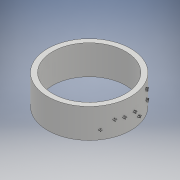
# Autodesk Inventor part: velky-vuz
Saved by Autodesk Inventor 2018 (Build 220112000, 112)
## iProperties
Created: 2019-09-09
Part Number: velky-vuz
Material: Generic
Document SubType Name: Modeling
Designer: dsikar
Density: 1 g/cm^3
Appearance: Default
Author: dsikar
Autodesk Inventor part; units mm, degrees
ref_plane "XZ Plane" through (0, 0, 0) normal (0, 1, 0) x (-1, 0, 0)
ref_plane "XY Plane" through (0, 0, 0) normal (0, 0, 1) x (1, 0, 0)
sketch "Sketch1" plane through (0, 0, 0) normal (0, 1, 0) x (-1, 0, 0)
  line L0 (8.7, 0) -> (9.9, 0)
  line L1 (9.9, 0) -> (9.9, 7)
  line L2 (9.9, 7) -> (8.7, 7)
  line L3 (8.7, 7) -> (8.7, 0)
  line L4 (0, -1.4) -> (0, 8.4) projected
  point P0 (0, 0)
  dimension "d0" = 1.2
  dimension "d1" = 7
  dimension "d2" = 8.7
  constraints: 8 end point, 2 parallel, 1 horizontal, 1 perpendicular
  measures "d0" distance of L2.end L1.end
  measures "d1" distance of L1.end L0.end
  measures "d2" distance from line of L3 point (0, 0)
revolve "Revolution1" add sketch "Sketch1" angle 360 about axis through (0, 0, -10) along (0, 0, 1)
ref_plane "Work Plane1" through (15, 0, 0) normal (1, 0, 0) x (0, 1, 0)
sketch "Sketch2" plane through (15, 0, 0) normal (1, 0, 0) x (0, 1, 0)
  line L0 (-6.8018, 10.1756) -> (6.3794, 10.1756) construction
  line L1 (6.3794, 10.1756) -> (6.3794, -3.0056) construction
  line L2 (6.3794, -3.0056) -> (-6.8018, -3.0056) construction
  line L3 (-6.8018, -3.0056) -> (-6.8018, 10.1756) construction
  line L4 (-5.9444, 2.3561) -> (-5.8589, 2.3561)
  line L5 (-5.8589, 1.9313) -> (-5.9444, 1.9313)
  line L6 (-5.6398, 2.2119) -> (-5.6398, 2.129)
  line L7 (-6.1956, 2.129) -> (-6.1956, 2.2119)
  line L8 (-3.4429, 4.0019) -> (-3.3959, 4.0019)
  line L9 (-3.3959, 3.4529) -> (-3.4429, 3.4529)
  line L10 (-3.0817, 3.7671) -> (-3.0817, 3.7274)
  line L11 (-3.721, 3.7274) -> (-3.721, 3.7671)
  line L12 (-1.532, 3.8011) -> (-1.483, 3.8011)
  line L13 (-1.483, 3.1927) -> (-1.532, 3.1927)
  line L14 (-1.1572, 3.556) -> (-1.1572, 3.51)
  line L15 (-1.829, 3.51) -> (-1.829, 3.556)
  line L16 (1.1865, 3.533) -> (1.1865, 3.4969)
  line L17 (0.5052, 3.4969) -> (0.5052, 3.533)
  line L18 (0.8159, 3.8011) -> (0.8688, 3.8011)
  line L19 (0.8688, 3.2117) -> (0.8159, 3.2117)
  line L20 (2.0208, 2.0898) -> (2.0975, 2.0898)
  line L21 (2.0975, 1.5943) -> (2.0208, 1.5943)
  line L22 (2.4219, 1.9313) -> (2.4219, 1.8421)
  line L23 (1.6905, 1.8421) -> (1.6905, 1.9313)
  line L24 (5.5222, 5.5708) -> (5.5222, 5.5026)
  line L25 (4.7754, 5.5026) -> (4.7754, 5.5708)
  line L26 (5.0253, 5.8028) -> (5.0939, 5.8028)
  line L27 (5.0939, 5.0977) -> (5.0253, 5.0977)
  line L28 (5.3072, 3.4529) -> (5.3766, 3.4529)
  line L29 (5.3766, 2.6743) -> (5.3072, 2.6743)
  line L30 (5.0253, 3.1061) -> (5.0253, 3.1927)
  line L31 (5.0253, 5.0977) -> (5.0253, 5.3948)
  line L32 (5.0253, 5.6103) -> (5.0253, 5.8028)
  line L33 (5.0939, 5.8028) -> (5.0939, 5.6303)
  line L34 (5.0939, 5.3748) -> (5.0939, 5.0977)
  arc A0 (4.9661, 5.5026) -> (5.0253, 5.3948) centre (5.0939, 5.5026) ccw
  arc A1 (5.0939, 5.3748) -> (5.2216, 5.5026) centre (5.0939, 5.5026) ccw
  line L35 (5.5222, 5.5026) -> (5.2216, 5.5026)
  line L36 (4.9661, 5.5026) -> (4.7754, 5.5026)
  line L37 (4.7754, 5.5708) -> (4.9859, 5.5708)
  line L38 (5.2018, 5.5708) -> (5.5222, 5.5708)
  arc A2 (5.2018, 5.5708) -> (5.0939, 5.6303) centre (5.0939, 5.5026) ccw
  arc A3 (5.0253, 5.6103) -> (4.9859, 5.5708) centre (5.0939, 5.5026) ccw
  line L39 (5.0253, 3.1927) -> (5.2596, 3.1927)
  line L40 (5.4936, 3.1927) -> (5.7458, 3.1927)
  line L41 (5.7458, 3.1061) -> (5.5222, 3.1061)
  line L42 (5.231, 3.1061) -> (5.0253, 3.1061)
  arc A4 (5.3072, 3.2341) -> (5.2596, 3.1927) centre (5.3766, 3.1061) ccw
  arc A5 (5.231, 3.1061) -> (5.3072, 2.9781) centre (5.3766, 3.1061) ccw
  line L43 (5.3072, 2.6743) -> (5.3072, 2.9781)
  line L44 (5.3072, 3.2341) -> (5.3072, 3.4529)
  line L45 (5.3766, 3.4529) -> (5.3766, 3.2517)
  line L46 (5.3766, 2.9605) -> (5.3766, 2.6743)
  arc A6 (5.3766, 2.9605) -> (5.5222, 3.1061) centre (5.3766, 3.1061) ccw
  arc A7 (5.4936, 3.1927) -> (5.3766, 3.2517) centre (5.3766, 3.1061) ccw
  line L47 (1.6905, 1.9313) -> (1.9625, 1.9313)
  line L48 (2.1667, 1.9313) -> (2.4219, 1.9313)
  line L49 (2.4219, 1.8421) -> (2.1823, 1.8421)
  line L50 (1.9469, 1.8421) -> (1.6905, 1.8421)
  arc A8 (2.0208, 1.9796) -> (1.9625, 1.9313) centre (2.0646, 1.8675) ccw
  arc A9 (1.9469, 1.8421) -> (2.0208, 1.7553) centre (2.0646, 1.8675) ccw
  line L51 (2.0208, 1.5943) -> (2.0208, 1.7553)
  line L52 (2.0208, 1.9796) -> (2.0208, 2.0898)
  line L53 (2.0975, 2.0898) -> (2.0975, 1.9833)
  line L54 (2.0975, 1.7516) -> (2.0975, 1.5943)
  arc A10 (2.0975, 1.7516) -> (2.1823, 1.8421) centre (2.0646, 1.8675) ccw
  arc A11 (2.1667, 1.9313) -> (2.0975, 1.9833) centre (2.0646, 1.8675) ccw
  line L55 (0.5052, 3.533) -> (0.6841, 3.533)
  line L56 (0.9948, 3.533) -> (1.1865, 3.533)
  line L57 (1.1865, 3.4969) -> (0.9959, 3.4969)
  line L58 (0.683, 3.4969) -> (0.5052, 3.4969)
  arc A12 (0.8159, 3.6652) -> (0.6841, 3.533) centre (0.8394, 3.51) ccw
  arc A13 (0.683, 3.4969) -> (0.8159, 3.3548) centre (0.8394, 3.51) ccw
  line L59 (0.8159, 3.2117) -> (0.8159, 3.3548)
  line L60 (0.8159, 3.6652) -> (0.8159, 3.8011)
  line L61 (0.8688, 3.8011) -> (0.8688, 3.6642)
  line L62 (0.8688, 3.3558) -> (0.8688, 3.2117)
  arc A14 (0.8688, 3.3558) -> (0.9959, 3.4969) centre (0.8394, 3.51) ccw
  arc A15 (0.9948, 3.533) -> (0.8688, 3.6642) centre (0.8394, 3.51) ccw
  line L63 (-1.1572, 3.51) -> (-1.3685, 3.51)
  line L64 (-1.6378, 3.51) -> (-1.829, 3.51)
  line L65 (-1.829, 3.556) -> (-1.6297, 3.556)
  line L66 (-1.3767, 3.556) -> (-1.1572, 3.556)
  arc A16 (-1.532, 3.6415) -> (-1.6297, 3.556) centre (-1.5032, 3.51) ccw
  arc A17 (-1.6378, 3.51) -> (-1.532, 3.3785) centre (-1.5032, 3.51) ccw
  line L67 (-1.532, 3.1927) -> (-1.532, 3.3785)
  line L68 (-1.532, 3.6415) -> (-1.532, 3.8011)
  line L69 (-1.483, 3.8011) -> (-1.483, 3.6431)
  line L70 (-1.483, 3.3769) -> (-1.483, 3.1927)
  arc A18 (-1.483, 3.3769) -> (-1.3685, 3.51) centre (-1.5032, 3.51) ccw
  arc A19 (-1.3767, 3.556) -> (-1.483, 3.6431) centre (-1.5032, 3.51) ccw
  line L71 (-3.3959, 4.0019) -> (-3.3959, 3.8762)
  line L72 (-3.4429, 3.8746) -> (-3.4429, 4.0019)
  line L73 (-3.721, 3.7671) -> (-3.5507, 3.7671)
  line L74 (-3.5531, 3.7274) -> (-3.721, 3.7274)
  line L75 (-3.4429, 3.4529) -> (-3.4429, 3.6031)
  line L76 (-3.3959, 3.6016) -> (-3.3959, 3.4529)
  line L77 (-3.0817, 3.7274) -> (-3.2768, 3.7274)
  line L78 (-3.2793, 3.7671) -> (-3.0817, 3.7671)
  arc A20 (-3.4429, 3.8746) -> (-3.5507, 3.7671) centre (-3.415, 3.7389) ccw
  arc A21 (-3.5531, 3.7274) -> (-3.4429, 3.6031) centre (-3.415, 3.7389) ccw
  arc A22 (-3.3959, 3.6016) -> (-3.2768, 3.7274) centre (-3.415, 3.7389) ccw
  arc A23 (-3.2793, 3.7671) -> (-3.3959, 3.8762) centre (-3.415, 3.7389) ccw
  line L79 (-5.6398, 2.129) -> (-5.7835, 2.129)
  line L80 (-6.0279, 2.129) -> (-6.1956, 2.129)
  line L81 (-6.1956, 2.2119) -> (-6.0232, 2.2119)
  line L82 (-5.7882, 2.2119) -> (-5.6398, 2.2119)
  arc A24 (-5.9444, 2.2846) -> (-6.0232, 2.2119) centre (-5.9057, 2.1636) ccw
  arc A25 (-6.0279, 2.129) -> (-5.9444, 2.0427) centre (-5.9057, 2.1636) ccw
  line L83 (-5.9444, 1.9313) -> (-5.9444, 2.0427)
  line L84 (-5.9444, 2.2846) -> (-5.9444, 2.3561)
  line L85 (-5.8589, 2.3561) -> (-5.8589, 2.2817)
  line L86 (-5.8589, 2.0456) -> (-5.8589, 1.9313)
  arc A26 (-5.8589, 2.0456) -> (-5.7835, 2.129) centre (-5.9057, 2.1636) ccw
  arc A27 (-5.7882, 2.2119) -> (-5.8589, 2.2817) centre (-5.9057, 2.1636) ccw
  line L87 (5.7458, 3.1927) -> (5.7458, 3.1061)
  point P0 (0, 0)
  constraints: 168 end point, 69 parallel, 56 point on circle, 28 centre point, 26 perpendicular, 21 horizontal, 1 vertical, 2 other
emboss "Emboss2" sketch "Sketch2" operation add depth 0.4 direction (1, 0, 0) wrap yes faces at (-9.7718, 1.5881, 2.3333)
body "Solid1"
